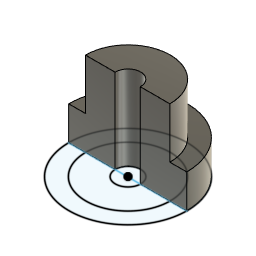
scpipi_plug v1 (Autodesk Fusion 360 design; units mm, degrees)
Autodesk Fusion 360 part; units mm, degrees
note: some values were not read from the file. Set by a fixed rule: which sketch regions a step uses.
sketch "Sketch1" plane through (0, 0, 0) normal (0, 0, 1) x (1, 0, 0)
  circle A0 centre (0, 0) radius 1.5
  circle A1 centre (0, 0) radius 5
  circle A2 centre (0, 0) radius 7
  line L0 (-6.9999, -0.039) -> (6.9999, -0.039)
  dimension "d1" = 3
  dimension "d2" = 10
  dimension "d3" = 14
  constraint coincident A0.centre A1.centre
  constraint concentric A0 A1
  constraint concentric A1 A2
  constraint coincident A2 L0.start
  constraint coincident A2 L0.end
  constraint horizontal L0
  measures "d1" diameter of A0
  measures "d2" diameter of A1
  measures "d3" diameter of A2
extrude "Extrude1" add sketch "Sketch1" along normal blind 10 contours A0 A1 L0 picked at (-1.1427, 3.6492)
extrude "Extrude2" add sketch "Sketch1" along normal blind 4 contours A1 A2 L0 picked at (-6.2922, 0.5587)
